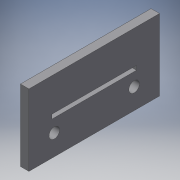
# Autodesk Inventor part: Part11
Saved by Autodesk Inventor 2016 (Build 200138000, 138)
## iProperties
Created: 2018-01-18
Part Number: Part11
Material: Generic
Document SubType Name: Modeling
Designer: student
Density: 1 g/cm^3
Appearance: Default
Author: student
Autodesk Inventor part; units mm, degrees
ref_plane "YZ Plane" through (0, 0, 0) normal (1, 0, 0) x (0, 1, 0)
ref_plane "XZ Plane" through (0, 0, 0) normal (0, 1, 0) x (-1, 0, 0)
ref_plane "XY Plane" through (0, 0, 0) normal (0, 0, 1) x (1, 0, 0)
sketch "Sketch1" plane through (0, 0, 0) normal (1, 0, 0) x (0, 1, 0)
  circle A0 centre (-39.4896, 239.2047) radius 4 projected
  circle A1 centre (-39.4896, 179.2047) radius 4 projected
  line L0 (-29.6646, 240.9547) -> (-29.6646, 177.4547) projected
  line L1 (-29.6646, 240.9547) -> (-26.4896, 240.9547) projected
  line L2 (-26.4896, 177.4547) -> (-26.4896, 240.9547) projected
  line L3 (-29.6646, 177.4547) -> (-26.4896, 177.4547) projected
  line L4 (-39.4896, 179.2047) -> (-29.6646, 179.2047) construction
  line L5 (-39.4896, 239.2047) -> (-29.6646, 239.2047) construction
  line L6 (-39.4896, 175.2047) -> (-39.4896, 243.2047) construction
  line L7 (-39.4896, 179.2047) -> (-39.4896, 160.1547) construction
  line L8 (-39.4896, 239.2047) -> (-39.4896, 258.2547) construction
  line L9 (-39.4896, 160.1547) -> (-1.3896, 160.1547) construction
  line L10 (-55.0646, 185.9297) -> (-55.0646, 179.5797) construction
  line L11 (-1.3896, 160.1547) -> (-55.0646, 160.1547)
  line L12 (-55.0646, 160.1547) -> (-55.0646, 258.2547)
  line L13 (-55.0646, 258.2547) -> (-1.3896, 258.2547)
  line L14 (-1.3896, 258.2547) -> (-1.3896, 160.1547)
  point P0 (0, 0)
  dimension "d0" = 63.5
  dimension "d1" = 3.175
  dimension "d2" = 68
  dimension "d3" = 9.825
  dimension "d4" = 19.05
  dimension "d5" = 19.05
  dimension "d6" = 38.1
  constraints: 20 end point, 4 perpendicular, 2 horizontal, 2 parallel, 2 point on line, 2 vertical, 2 vertical alignment, 2 other
  measures "d0" distance of L2.start L1.end
  measures "d1" distance of L0.end L2.start
  measures "d2" distance of L6.start L6.end
  measures "d3" distance of L5.start L5.end
  measures "d4" distance of L4.start L7.end
  measures "d5" distance of L5.start L8.end
  measures "d6" distance of L7.end L9.end
extrude "Extrusion1" add sketch "Sketch1" along normal blind 6.35
body "Solid1"
